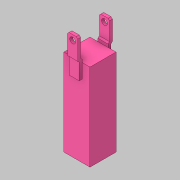
# Autodesk Inventor part: B6-A2
Saved by Autodesk Inventor 2018.1 (Build 221171000, 171)
## iProperties
Created: 2018-06-23
Part Number: B6-A2
Material: Všeobecné
Document SubType Name: Modeling
Designer: PS
Density: 1 g/cm^3
Appearance: Výchozí
Author: PS
Autodesk Inventor part; units mm, degrees
ref_plane "YZ Plane" through (0, 0, 0) normal (1, 0, 0) x (0, 1, 0)
ref_plane "XZ Plane" through (0, 0, 0) normal (0, 1, 0) x (-1, 0, 0)
ref_plane "XY Plane" through (0, 0, 0) normal (0, 0, 1) x (1, 0, 0)
sketch "Náčrt1" plane through (0, 0, 0) normal (0, 0, 1) x (1, 0, 0)
  line L0 (-90, -90) -> (90, -90)
  line L1 (90, -90) -> (90, 90)
  line L2 (90, 90) -> (-90, 90)
  line L3 (-90, 90) -> (-90, -90)
  line L4 (-90, -90) -> (90, 90) construction
  line L5 (90, -90) -> (-90, 90) construction
  point P0 (0, 0)
  dimension "d0" = 180
  constraints: 12 end point, 2 midpoint, 2 parallel, 2 perpendicular, 1 horizontal
  measures "d0" distance of L1.end L2.end
extrude "Vysunutí1" add sketch "Náčrt1" along normal blind 600
sketch "Náčrt2" plane through (0, 0, 0) normal (1, 0, 0) x (0, 1, 0)
  line L0 (-90, 0) -> (-90, 600) projected
  line L1 (-100, 630) -> (-100, 765)
  line L2 (-120, 681.7157) -> (-120, 540)
  line L3 (-90, 600) -> (90, 600) projected
  line L4 (0, 600) -> (0, 773.8359) construction
  line L5 (-90, 0) -> (90, 0) projected
  line L6 (-90, 500) -> (-90, 620)
  line L7 (-90, 620) -> (-100, 630)
  line L8 (-120, 765) -> (-120, 621.7157)
  line L9 (-120, 621.7157) -> (-110, 611.7157)
  line L10 (-110, 611.7157) -> (-110, 500)
  line L11 (-120, 765) -> (-100, 765)
  line L12 (-110, 500) -> (-90, 500)
  line L13 (-120, 730) -> (-100, 730) construction
  point P0 (0, 0)
  dimension "d5" = 100
  dimension "d22" = 135
  dimension "d24" = 20
  dimension "d26" = 20
  dimension "d35" = 35
  dimension "d36" = 130
  dimension "d37" = 100
  constraints: 22 end point, 4 point on line, 2 horizontal, 1 midpoint, 1 perpendicular, 1 vertical, 2 other
  measures "d5" distance between parallel lines of L1 L4
  measures "d22" angle of L1 L7
  measures "d24" distance between parallel lines of L1 L8
  measures "d26" distance from line of L3 L6.end
  measures "d35" distance between parallel lines of L13 L11
  measures "d36" distance between parallel lines of L3 L13
  measures "d37" distance from line of L12 L0.end
extrude "Vysunutí2" add sketch "Náčrt2" along normal mid plane 70
sketch "Náčrt3" plane through (-30, -120, 582.0978) normal (0, -1, 0) x (1, 0, 0)
  line L0 (-5, 182.9022) -> (65, 182.9022) projected
  line L1 (30, 182.9022) -> (30, 119.5637) construction
  circle A0 centre (30, 147.9022) radius 20
  point P0 (30, -582.0978)
  dimension "d11" = 40
  dimension "d12" = 35
  dimension "d25" = 70
  constraints: 2 end point, 1 centre point, 1 midpoint, 1 point on line, 1 vertical
  measures "d11" diameter of A0
  measures "d12" distance from line of A0.centre L0
  measures "d25" distance of L0.start L0.end
extrude "Vysunutí3" cut sketch "Náčrt3" against normal blind 60
chamfer "Zkosení1" distance 10 angle 45 2 edges at (35, -110, 765) (-35, -110, 765)
mirror "Zrcadlit1" about plane through (0, 0, 0) normal (0, 1, 0)
sketch "Náčrt5" plane through (0, 0, 0) normal (0, 0, -1) x (-1, 0, 0)
  circle A0 centre (0, 0) radius 65
  dimension "d40" = 130
  constraints: 1 centre point, 1 coincident
  measures "d40" diameter of A0
extrude "Vysunutí5" add sketch "Náčrt5" along normal blind 20
equation "\"d12\" = 0.5 * d25"
